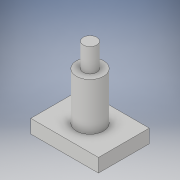
# Autodesk Inventor part: LaserMountMount
Saved by Autodesk Inventor 2019 (Build 230136000, 136)
## iProperties
Created: 2019-05-18
Part Number: LaserMountMount
Material: Generic
Document SubType Name: Modeling
Designer: Henry
Density: 1 g/cm^3
Appearance: Default
Author: Henry
Autodesk Inventor part; units mm, degrees
ref_plane "YZ Plane" through (0, 0, 0) normal (1, 0, 0) x (0, 1, 0)
ref_plane "XZ Plane" through (0, 0, 0) normal (0, 1, 0) x (-1, 0, 0)
ref_plane "XY Plane" through (0, 0, 0) normal (0, 0, 1) x (1, 0, 0)
sketch "Sketch1" plane through (0, 0, 0) normal (0, 1, 0) x (-1, 0, 0)
  line L0 (0, 0) -> (10, 0)
  line L1 (10, 0) -> (10, -7.5)
  line L2 (10, -7.5) -> (0, -7.5)
  line L3 (0, -7.5) -> (0, 0)
  dimension "d0" = 10
  dimension "d1" = 7.5
  constraints: 8 end point, 2 parallel, 1 horizontal, 1 perpendicular
  measures "d0" distance of L1.end L2.end
  measures "d1" distance of L0.end L1.end
extrude "Extrusion1" add sketch "Sketch1" along normal blind 2
sketch "Sketch2" plane through (0, 2, 0) normal (0, 1, 0) x (1, 0, 0)
  line L0 (-10, 7.5) -> (-10, 0) projected
  line L1 (-10, 0) -> (-5, 0)
  line L2 (-5, 0) -> (-5, 3.75)
  line L3 (-5, 3.75) -> (-10, 3.75)
  line L4 (-10, 3.75) -> (-10, 0)
  circle A0 centre (-5, 3.75) radius 2
  point P0 (0, 0)
  dimension "d4" = 5
  dimension "d5" = 3.75
  dimension "d6" = 4
  constraints: 8 end point, 2 parallel, 1 centre point, 1 coincident, 1 horizontal, 1 perpendicular
  measures "d4" distance of L3.end L2.end
  measures "d5" distance of L2.end L1.end
  measures "d6" diameter of A0
extrude "Extrusion2" add sketch "Sketch2" along normal blind 7 contours A0 L2 L3 | L3 L2 A0
sketch "Sketch3" plane through (-5, 9, -3.75) normal (0, 1, 0) x (1, 0, 0)
  circle A0 centre (0, 0) radius 1
  point P0 (5, -3.75)
  dimension "d9" = 2
  constraints: 1 centre point
  measures "d9" diameter of A0
extrude "Extrusion3" add sketch "Sketch3" along normal blind 3.5
body "Solid1"
